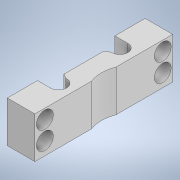
# Autodesk Inventor part: YCarriageFrontHolder
Saved by Autodesk Inventor 2020 (Build 240168000, 168)
## iProperties
Created: 2022-04-26
Part Number: YCarriageFrontHolder
Material: Ogólny
Document SubType Name: Modeling
Designer: mikoma
Density: 1 g/cm^3
Appearance: Domyślna
Author: mikoma
Autodesk Inventor part; units mm, degrees
ref_plane "YZ Plane" through (0, 0, 0) normal (1, 0, 0) x (0, 1, 0)
ref_plane "XZ Plane" through (0, 0, 0) normal (0, 1, 0) x (-1, 0, 0)
ref_plane "XY Plane" through (0, 0, 0) normal (0, 0, 1) x (1, 0, 0)
sketch "Szkic2" plane through (0, 0, 0) normal (0, 1, 0) x (-1, 0, 0)
  line L0 (-5, 13) -> (-5, -13)
  line L1 (1, -20.25) -> (1, 20.25)
  line L2 (-8.0627, 14.7682) -> (-5, 13)
  line L3 (-5, 16.0869) -> (-5, 13) construction
  arc A0 (-8.0627, 14.7682) -> (-5, 16.0869) centre (-8.5, 20) ccw construction
  line L4 (-3.256, 20.25) -> (-5, 20.25) construction
  arc A1 (-5, 16.0869) -> (-3.256, 20.25) centre (-8.5, 20) ccw construction
  line L5 (1, 20.25) -> (-3.256, 20.25)
  line L6 (-5, 20.25) -> (-5, 16.0869) construction
  line L7 (-5, -13) -> (-8.0627, -14.7682)
  line L8 (-5, -13) -> (-5, -16.0869) construction
  arc A2 (-5, -16.0869) -> (-8.0627, -14.7682) centre (-8.5, -20) ccw construction
  line L9 (-3.256, -20.25) -> (1, -20.25)
  arc A3 (-3.256, -20.25) -> (-5, -16.0869) centre (-8.5, -20) ccw construction
  line L10 (-5, -16.0869) -> (-5, -20.25) construction
  line L11 (-5, -20.25) -> (-3.256, -20.25) construction
  arc A4 (-8.0627, -14.7682) -> (-3.256, -20.25) centre (-8.5, -20) ccw
  arc A5 (-3.256, 20.25) -> (-8.0627, 14.7682) centre (-8.5, 20) ccw
  line L12 (0, 45) -> (-18, 45)
  line L13 (-18, 45) -> (-18, -45)
  line L14 (-18, -45) -> (0, -45)
  line L15 (0, -45) -> (0, 45)
  line L16 (-8.5, 25.25) -> (0, 25.25)
  line L17 (-8.5, -25.25) -> (0, -25.25)
  point P0 (0, 0)
  point P1 (0, -20.25)
  point P2 (0, 20.25)
  dimension "d0" = 10.5
  dimension "d1" = 6
  dimension "d2" = 3.5
  dimension "d3" = 120
  dimension "d4" = 120
  dimension "d5" = 26
  dimension "d6" = 40
  dimension "d8" = 7
  dimension "d9" = 0.25
  dimension "d10" = 0.25
  dimension "d12" = 9.5
  dimension "d14" = 1
  dimension "d15" = 20
  dimension "d16" = 90
  dimension "d17" = 45
  dimension "d18" = 18
  constraints: 36 end point, 14 point on circle, 9 parallel, 6 centre point, 5 perpendicular, 2 horizontal, 2 point on line, 2 tangent, 1 equal radius, 1 vertical alignment
  measures "d0" diameter of A2
  measures "d1" distance of L10.end L1.start
  measures "d2" distance from line of L6 A2.centre
  measures "d3" angle of L2 L3
  measures "d4" angle of L3 L7
  measures "d5" distance of L0.start L0.end
  measures "d6" distance of A0.centre A2.centre
  measures "d8" vertical distance of A0.centre L0.start
  measures "d9" distance from line of L5 A0.centre
  measures "d10" distance from line of L9 A2.centre
  measures "d12" distance from line of L1 A0.centre
  measures "d14" distance from line of L1 point (0, 0)
  measures "d15" vertical distance of A0.centre point (0, 0)
  measures "d16" distance of L12.end L13.end
  measures "d17" distance from line of point (0, 0) L14
  measures "d18" distance of L13.end L14.end
extrude "Wyciągnięcie proste1" add sketch "Szkic2" along normal blind 27 contours L0 L7 A4 L17 L15 L14 L13 L12 L16 A5 L2
sketch "Szkic3" plane through (18, 0, 45) normal (1, 0, 0) x (0, 0, -1)
  circle A0 centre (6.5, 20.5) radius 3.25
  circle A1 centre (6.5, 8.5) radius 3.25
  circle A2 centre (83.5, 20.5) radius 3.25
  circle A3 centre (83.5, 8.5) radius 3.25
  line L0 (0, 0) -> (0, 27) projected
  line L1 (0, 27) -> (90, 27) projected
  line L2 (90, 0) -> (90, 27) projected
  circle A4 centre (6.5, 20.5) radius 5.5
  circle A5 centre (6.5, 8.5) radius 5.5
  circle A6 centre (83.5, 20.5) radius 5.5
  circle A7 centre (83.5, 8.5) radius 5.5
  point P0 (45, 0)
  dimension "d21" = 6.5
  dimension "d22" = 6.5
  dimension "d23" = 6.5
  dimension "d24" = 12
  dimension "d25" = 6.5
  dimension "d26" = 11
  constraints: 8 centre point, 6 equal radius, 4 coincident, 2 horizontal alignment, 2 vertical alignment
  measures "d21" diameter of A0
  measures "d22" distance from line of L0 A0.centre
  measures "d23" distance from line of L1 A0.centre
  measures "d24" distance of A1.centre A0.centre
  measures "d25" distance from line of L2 A2.centre
  measures "d26" diameter of A4
extrude "Wyciągnięcie proste2" cut sketch "Szkic3" against normal through all contours A0 | A1 | A2 | A3
extrude "Wyciągnięcie proste3" cut sketch "Szkic3" against normal blind 8 contours A1 | A2 | A3 | A4 | A5 | A6 | A7
sketch "Szkic4" plane through (0, 27, 0) normal (0, 1, 0) x (1, 0, 0)
  line L0 (18, -45) -> (18, 45) projected
  circle A0 centre (38.5, 0) radius 22
  point P0 (0, 0)
  dimension "d34" = 44
  dimension "d37" = 20.5
  constraints: 1 centre point, 1 horizontal alignment
  measures "d34" diameter of A0
  measures "d37" distance from line of L0 A0.centre
extrude "Wyciągnięcie proste4" cut sketch "Szkic4" against normal through all
